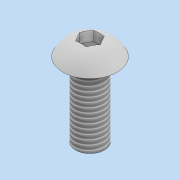
# Autodesk Inventor part: Screw
Saved by Autodesk Inventor 2022 (Build 260153000, 153)
## iProperties
Created: 2023-02-12
Part Number: Screw
Material: Generic
Document SubType Name: Modeling
Designer: coled
Density: 1 g/cm^3
Appearance: Default
Author: coled
Autodesk Inventor part; units mm, degrees
ref_plane "YZ Plane" through (0, 0, 0) normal (1, 0, 0) x (0, 1, 0)
ref_plane "XZ Plane" through (0, 0, 0) normal (0, 1, 0) x (-1, 0, 0)
ref_plane "XY Plane" through (0, 0, 0) normal (0, 0, 1) x (1, 0, 0)
sketch "Sketch1" plane through (0, 0, 0) normal (1, 0, 0) x (0, 1, 0)
  line L0 (0, 0) -> (0, -4.7)
  line L1 (0, 0) -> (3, 0)
  arc A0 (0, -4.7) -> (3, 0) centre (-2.1737, -0.0051) ccw
  dimension "d0" = 4.7
  dimension "d1" = 3
  constraints: 4 end point, 2 point on circle, 1 centre point, 1 horizontal, 1 vertical
  measures "d0" distance of L0.start L0.end
  measures "d1" distance of L0.start L1.end
revolve "Revolution1" add sketch "Sketch1" angle 360 about axis through (0, 0, 0) along (0, 1, 0)
sketch "Sketch2" plane through (0, 0, 0) normal (0, -1, 0) x (1, 0, 0)
  circle A0 centre (0, 0) radius 2.5
  dimension "d3" = 5
  constraints: 1 centre point, 1 coincident
  measures "d3" diameter of A0
extrude "Extrusion1" add sketch "Sketch2" along normal blind 12.8
thread "Thread1" size "M5x0.8" class "6g" standard "ANSI Metric M Profile" full length
ref_plane "Work Plane1" through (0, 3, 0) normal (0, -1, 0) x (1, 0, 0)
sketch "Sketch3" plane through (0, 3, 0) normal (0, -1, 0) x (1, 0, 0)
  line L0 (0, 0) -> (0, -1.575)
  circle A0 centre (0, 0) radius 2.5 projected
  line L1 (-0.9093, -1.575) -> (-1.8187, 0)
  line L2 (-1.8187, 0) -> (-0.9093, 1.575)
  line L3 (-0.9093, 1.575) -> (0.9093, 1.575)
  line L4 (0.9093, 1.575) -> (1.8187, 0)
  line L5 (1.8187, 0) -> (0.9093, -1.575)
  line L6 (0.9093, -1.575) -> (-0.9093, -1.575)
  dimension "d9" = 1.575
  constraints: 14 end point, 1 coincident, 1 midpoint, 1 vertical, 13 other
  measures "d9" distance of L0.start L0.end
extrude "Extrusion2" cut sketch "Sketch3" along normal blind 2 contours L1 L2 L3 L4 L5 L6
body "Solid1"
